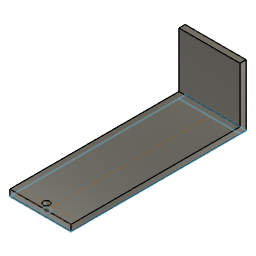
Power Supply Lock v8 (Autodesk Fusion 360 design; units mm, degrees)
Autodesk Fusion 360 part; units mm, degrees
sketch "Schizzo1" plane through (0, 0, 0) normal (0, 0, 1) x (1, 0, 0)
  line L0 (37.9329, 75.2335) -> (67.9329, 75.2335)
  line L1 (67.9329, 75.2335) -> (67.9329, -10.7665)
  line L2 (67.9329, -10.7665) -> (37.9329, -10.7665)
  line L3 (37.9329, -10.7665) -> (37.9329, 75.2335)
  line L4 (37.9329, -7.7665) -> (67.9329, -7.7665) construction
  line L5 (52.9329, 75.2335) -> (52.9329, -10.7665) construction
  line L6 (37.9329, 72.2335) -> (67.9329, 72.2335)
  circle A0 centre (52.9329, -7.7665) radius 1.6
  line L7 (37.9329, -4.7665) -> (67.9329, -4.7665) construction
  dimension "d1" = 30
  dimension "d3" = 3
  dimension "d4" = 3
  dimension "d5" = 3.2
  dimension "d13" = 6
  dimension "d14" = 77
  constraint horizontal L0
  constraint vertical L1
  constraint horizontal L2
  constraint vertical L3
  constraint coincident L3 L4.start
  constraint coincident L1 L4.end
  constraint perpendicular L1 L4
  constraint midpoint L0 L5.start
  constraint midpoint L2 L5.end
  constraint coincident L3 L6.start
  constraint coincident L1 L6.end
  constraint perpendicular L1 L6
  constraint midpoint L4 A0.centre
  constraint coincident L3 L7.start
  constraint coincident L1 L7.end
  constraint perpendicular L1 L7
  measures "d1" distance of L0.start L0.end
  measures "d3" distance of L2 L4
  measures "d4" distance of L0 L6
  measures "d5" diameter of A0
  measures "d13" distance of L2 L7
  measures "d14" distance of L6 L7
extrude "Estrusione1" add sketch "Schizzo1" along normal blind 3 contours L1 L2 L3 L6
extrude "Estrusione2" add sketch "Schizzo1" along normal blind 30 contours L0 L1 L3 L6
